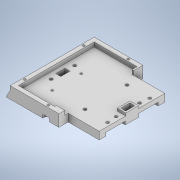
# Autodesk Inventor part: jeff
Saved by Autodesk Inventor 2020 (Build 240168000, 168)
## iProperties
Created: 2023-02-07
Part Number: jeff
Material: Generic
Document SubType Name: Modeling
Designer: user
Density: 1 g/cm^3
Appearance: Default
Author: user
Autodesk Inventor part; units mm, degrees
ref_plane "YZ Plane" through (0, 0, 0) normal (1, 0, 0) x (0, 1, 0)
ref_plane "XZ Plane" through (0, 0, 0) normal (0, 1, 0) x (-1, 0, 0)
ref_plane "XY Plane" through (0, 0, 0) normal (0, 0, 1) x (1, 0, 0)
sketch "Sketch1" plane through (0, 0, 0) normal (0, 1, 0) x (-1, 0, 0)
  line L0 (0, 0) -> (-100, 0)
  line L1 (-100, 0) -> (-100, -100)
  line L2 (-100, -100) -> (0, -100)
  line L3 (0, -100) -> (0, 0)
  dimension "d0" = 100
  dimension "d1" = 100
  constraints: 8 end point, 2 parallel, 1 horizontal, 1 perpendicular
  measures "d0" distance of L2.end L1.end
  measures "d1" distance of L1.end L0.end
extrude "base" add sketch "Sketch1" along normal blind 9
sketch "Sketch2" plane through (0, 9, 0) normal (0, 1, 0) x (1, 0, 0)
  circle A0 centre (96, 25) radius 1.75
  line L0 (100, 0) -> (100, 100) projected
  circle A1 centre (69, 25) radius 1.75
  line L1 (0, 0) -> (100, 0) projected
  line L2 (100, 50) -> (95, 50)
  circle A2 centre (96, 75) radius 1.75
  circle A3 centre (69, 75) radius 1.75
  line L3 (63, 0) -> (63, 100)
  line L4 (100, 100) -> (0, 100) projected
  line L5 (100, 25) -> (100, 11)
  line L6 (100, 11) -> (63, 11)
  line L7 (100, 89) -> (63, 89)
  circle A4 centre (82, 25) radius 17.5
  point P0 (63, 89)
  dimension "d6" = 4
  dimension "d7" = 3.5
  dimension "d9" = 3.5
  dimension "d10" = 27
  dimension "d11" = 25
  dimension "d13" = 37
  dimension "d14" = 14
  dimension "d17" = 35
  constraints: 10 end point, 5 centre point, 5 point on line, 4 symmetric about line, 1 horizontal, 1 horizontal alignment, 1 midpoint, 1 perpendicular, 1 vertical, 2 other
  measures "d6" distance from line of L0 A0.centre
  measures "d7" diameter of A0
  measures "d9" diameter of A1
  measures "d10" distance of A0.centre A1.centre
  measures "d11" distance from line of L1 A0.centre
  measures "d13" distance between parallel lines of L0 L3
  measures "d14" distance of L5.start L5.end
  measures "d17" diameter of A4
extrude "wheel space" cut sketch "Sketch2" against normal through all contours A0 | L1 L3 L6 A4 L0 | A4 L6 | L3 L4 L0 L7 | A1 | A2 | A3 picked at (84.4264, 10.3619)
sketch "Sketch3" plane through (0, 0, 0) normal (0, 0, 1) x (1, 0, 0)
  line L0 (63, 9) -> (0, 9) projected
  line L1 (0, 0) -> (0, 9) projected
  line L2 (63, 0) -> (0, 0) projected
  line L3 (5, 9) -> (0, 0)
  dimension "d18" = 5
  constraints: 2 end point, 1 point on line
  measures "d18" distance from line of L1 L3.start
extrude "ramp" cut sketch "Sketch3" against normal through all
sketch "Sketch4" plane through (0, 9, 0) normal (0, 1, 0) x (1, 0, 0)
  circle A0 centre (69, 75) radius 1.75 projected
  circle A1 centre (96, 25) radius 1.75 projected
  circle A2 centre (96, 75) radius 1.75 projected
  circle A3 centre (69, 25) radius 1.75 projected
  line L0 (5, 100) -> (5, 0) projected
  line L1 (5, 0) -> (63, 0) projected
  line L2 (63, 0) -> (63, 11) projected
  line L3 (63, 11) -> (100, 11) projected
  line L4 (100, 11) -> (100, 89) projected
  line L5 (100, 89) -> (63, 89) projected
  line L6 (63, 89) -> (63, 100) projected
  line L7 (63, 100) -> (5, 100) projected
  line L8 (63, 100) -> (63, 89) projected
  line L9 (61, 95) -> (10, 95)
  line L10 (10, 95) -> (10, 5)
  line L11 (10, 5) -> (63, 5)
  line L12 (63, 11) -> (63, 0) projected
  line L13 (63, 89) -> (61, 89)
  line L14 (61, 89) -> (61, 95)
  line L15 (63, 5) -> (53, 5)
  line L16 (53, 5) -> (53, 7)
  line L17 (53, 7) -> (63, 7)
  line L18 (63, 7) -> (63, 5)
  point P0 (0, 0)
  point P1 (63, 95)
  dimension "d21" = 5
  dimension "d22" = 5
  dimension "d23" = 5
  dimension "d64" = 2
  dimension "d72" = 10
  dimension "d73" = 2
  constraints: 18 end point, 5 perpendicular, 2 horizontal, 2 parallel, 1 point on line
  measures "d21" distance between parallel lines of L11 L1
  measures "d22" distance between parallel lines of L0 L10
  measures "d23" distance between parallel lines of L7 L9
  measures "d64" distance of L5.end L13.end
  measures "d72" distance of L16.end L17.end
  measures "d73" distance of L15.end L16.end
extrude "walls" add sketch "Sketch4" along normal blind 5 contours L7 L6 L13 L14 L9 L10 L11 L2 L1 L0 | L11 L16 L17 L2
sketch "Sketch5" plane through (0, 9, 0) normal (0, 1, 0) x (1, 0, 0)
  line L0 (22.7322, 84.5) -> (12.7322, 84.5)
  line L1 (12.7322, 84.5) -> (12.7322, 44.5)
  line L2 (12.7322, 44.5) -> (22.7322, 44.5)
  line L3 (22.7322, 44.5) -> (22.7322, 84.5)
  line L4 (14.7322, 44.5) -> (20.7322, 44.5)
  line L5 (20.7322, 44.5) -> (20.7322, 55.5)
  line L6 (20.7322, 55.5) -> (14.7322, 55.5)
  line L7 (14.7322, 55.5) -> (14.7322, 44.5)
  line L8 (14.7322, 44.5) -> (20.7322, 55.5) construction
  line L9 (20.7322, 44.5) -> (14.7322, 55.5) construction
  line L10 (10, 5) -> (10, 95) projected
  circle A0 centre (17.7322, 64) radius 1.75
  line L11 (100, 84.5) -> (90, 84.5)
  line L12 (90, 84.5) -> (90, 44.5)
  line L13 (90, 44.5) -> (100, 44.5)
  line L14 (100, 44.5) -> (100, 84.5)
  line L15 (92, 44.5) -> (98, 44.5)
  line L16 (98, 44.5) -> (98, 55.5)
  line L17 (98, 55.5) -> (92, 55.5)
  line L18 (92, 55.5) -> (92, 44.5)
  line L19 (92, 44.5) -> (98, 55.5) construction
  line L20 (98, 44.5) -> (92, 55.5) construction
  circle A1 centre (95, 64) radius 1.75
  circle A2 centre (96, 75) radius 1.75 projected
  line L21 (100, 11) -> (100, 89) projected
  circle A3 centre (95, 36) radius 1.75
  circle A4 centre (17.7322, 36) radius 1.75
  line L22 (100, 57.5) -> (90, 57.5)
  line L23 (90, 57.5) -> (90, 42.5)
  line L24 (90, 42.5) -> (100, 42.5)
  line L25 (100, 42.5) -> (100, 57.5)
  line L26 (100, 57.5) -> (90, 42.5) construction
  line L27 (90, 57.5) -> (100, 42.5) construction
  point P0 (0, 0)
  point P1 (17.7322, 50)
  point P2 (10, 50)
  point P3 (17.7322, 50)
  point P4 (95, 50)
  point P5 (95, 50)
  point P6 (95, 50)
  point P7 (17.7322, 50)
  point P8 (92, 44.5)
  point P9 (98, 44.5)
  point P10 (95, 84.5)
  dimension "d26" = 10
  dimension "d27" = 40
  dimension "d28" = 5.5
  dimension "d29" = 6
  dimension "d30" = 11
  dimension "d31" = 3.5
  dimension "d32" = 14
  dimension "d33" = 10
  dimension "d34" = 40
  dimension "d35" = 5.5
  dimension "d36" = 6
  dimension "d37" = 11
  dimension "d38" = 3.5
  dimension "d39" = 14
  dimension "d60" = 3.5
  dimension "d61" = 14
  dimension "d62" = 3.5
  dimension "d63" = 14
  dimension "d65" = 10
  dimension "d66" = 15
  constraints: 52 end point, 12 midpoint, 9 parallel, 5 horizontal, 5 perpendicular, 4 centre point, 1 collinear, 1 horizontal alignment, 1 vertical alignment
  measures "d26" distance of L2.end L1.end
  measures "d27" distance of L1.end L0.end
  measures "d28" distance from line of L2 point (17.732, 50)
  measures "d29" distance of L6.end L5.end
  measures "d30" distance of L5.end L4.end
  measures "d31" diameter of A0
  measures "d32" distance of point (17.732, 50) A0.centre
  measures "d33" distance of L14.start L12.end
  measures "d34" distance of L12.end L12.start
  measures "d35" distance from line of L13 point (95, 50)
  measures "d36" distance of L17.end L16.end
  measures "d37" distance of L16.end L15.end
  measures "d38" diameter of A1
  measures "d39" distance of point (95, 50) A1.centre
  measures "d60" diameter of A3
  measures "d61" distance of point (95, 50) A3.centre
  measures "d62" diameter of A4
  measures "d63" distance of A4.centre point (17.732, 50)
  measures "d65" distance of L24.end L23.end
  measures "d66" distance of L23.end L22.end
extrude "ir sensor" cut sketch "Sketch5" against normal through all contours L2 L7 L6 L5 | A0 | L13 L18 L17 L16 | A1 | A3 | A4
sketch "Sketch8" plane through (0, 14, 0) normal (0, 1, 0) x (1, 0, 0)
  line L0 (61, 89) -> (63, 89) projected
  line L1 (63, 89) -> (63, 100) projected
  line L2 (63, 100) -> (5, 100) projected
  line L3 (5, 100) -> (5, 0) projected
  line L4 (5, 0) -> (63, 0) projected
  line L5 (63, 0) -> (63, 7) projected
  line L6 (63, 7) -> (53, 7) projected
  line L7 (53, 7) -> (53, 5) projected
  line L8 (53, 5) -> (10, 5) projected
  line L9 (10, 5) -> (10, 95) projected
  line L10 (10, 95) -> (61, 95) projected
  line L11 (61, 95) -> (61, 89) projected
  circle A0 centre (7.5, 85) radius 1.25
  circle A1 centre (7.5, 15) radius 1.25
  circle A2 centre (48, 2.5) radius 1.25
  circle A3 centre (48, 97.5) radius 1.25
  point P0 (0, 0)
  dimension "d82" = 2.5
  dimension "d84" = 2.5
  dimension "d85" = 2.5
  dimension "d87" = 2.5
  dimension "d88" = 15
  dimension "d89" = 15
  dimension "d90" = 15
  dimension "d91" = 2.5
  dimension "d92" = 2.5
  dimension "d93" = 2.5
  constraints: 4 centre point, 2 vertical alignment
  measures "d82" diameter of A0
  measures "d84" diameter of A1
  measures "d85" diameter of A2
  measures "d87" diameter of A3
  measures "d88" distance from line of L2 A0.centre
  measures "d89" distance from line of L4 A1.centre
  measures "d90" distance from line of L1 A3.centre
  measures "d91" distance from line of L3 A0.centre
  measures "d92" distance from line of L10 A3.centre
  measures "d93" distance from line of L4 A2.centre
sketch "Sketch6" plane through (0, 9, 0) normal (0, 1, 0) x (1, 0, 0)
  line L0 (20.7322, 44.5) -> (14.7322, 44.5) projected
  circle A0 centre (17.7322, 64) radius 1.75 projected
  line L1 (53, 5) -> (10, 5) projected
  line L2 (10, 95) -> (61, 95) projected
  circle A1 centre (69, 25) radius 1.75 projected
  circle A2 centre (96, 25) radius 1.75 projected
  circle A3 centre (69, 25) radius 1.75 projected
  circle A4 centre (96, 25) radius 1.75 projected
  line L3 (69, 25) -> (96, 25)
  circle A5 centre (30, 25) radius 1.25
  line L4 (10, 5) -> (10, 95) projected
  circle A6 centre (30, 59.5) radius 1.25
  circle A7 centre (48, 97.5) radius 1.25 projected
  circle A8 centre (48, 2.5) radius 1.25 projected
  circle A9 centre (7.5, 85) radius 1.25 projected
  circle A10 centre (7.5, 15) radius 1.25 projected
  point P0 (0, 0)
  point P1 (63, 5)
  point P2 (63, 95)
  dimension "d75" = 2.5
  dimension "d76" = 20
  dimension "d77" = 20
  dimension "d79" = 2.5
  dimension "d80" = 34.5
  constraints: 2 centre point, 2 end point, 1 horizontal
  measures "d75" diameter of A5
  measures "d76" distance from line of L1 A5.centre
  measures "d77" distance from line of L4 A5.centre
  measures "d79" diameter of A6
  measures "d80" distance of A5.centre A6.centre
extrude "mount holes" cut sketch "Sketch6" against normal through all both and the other way through all contours A5 | A6 | A7 | A8 | A9 | A10
sketch "Sketch7" plane through (0, 0, 0) normal (0, -1, 0) x (1, 0, 0)
  line L0 (92, -44.5) -> (98, -44.5) projected
  line L1 (98, -44.5) -> (98, -55.5) projected
  line L2 (98, -55.5) -> (92, -55.5) projected
  line L3 (92, -55.5) -> (92, -44.5) projected
  circle A0 centre (17.7322, -64) radius 1.75 projected
  circle A1 centre (95, -64) radius 1.75 projected
  line L4 (20.7322, -44.5) -> (20.7322, -55.5) projected
  line L5 (20.7322, -55.5) -> (14.7322, -55.5) projected
  line L6 (14.7322, -55.5) -> (14.7322, -44.5) projected
  line L7 (14.7322, -44.5) -> (20.7322, -44.5) projected
  circle A2 centre (69, -75) radius 1.75 projected
  circle A3 centre (96, -25) radius 1.75 projected
  circle A4 centre (96, -75) radius 1.75 projected
  circle A5 centre (69, -25) radius 1.75 projected
  line L8 (63, -100) -> (63, -89) projected
  line L9 (63, -89) -> (100, -89) projected
  line L10 (100, -11) -> (100, -89) projected
  line L11 (100, -11) -> (63, -11) projected
  line L12 (63, -11) -> (63, 0) projected
  line L13 (0, 0) -> (63, 0) projected
  line L14 (0, -100) -> (0, 0) projected
  line L15 (63, -100) -> (0, -100) projected
  circle A6 centre (69, -75) radius 6
  circle A7 centre (69, -25) radius 1.75 projected
  circle A8 centre (69, -25) radius 6
  circle A9 centre (96, -25) radius 1.75 projected
  circle A10 centre (17.7322, -64) radius 6
  circle A11 centre (95, -36) radius 1.75 projected
  arc A12 (89, -36) -> (95, -42) centre (95, -36) ccw
  line L16 (98, -31) -> (98.3166, -31)
  line L17 (100, -11) -> (100, -89) projected
  line L18 (96, -19) -> (100, -19)
  line L19 (100, -50) -> (98.3161, -50)
  line L20 (95, -42) -> (100, -42)
  circle A13 centre (17.7322, -36) radius 1.75 projected
  circle A14 centre (17.7322, -36) radius 6
  line L21 (92, -19) -> (96, -19)
  line L22 (89, -36) -> (89, -19)
  line L23 (89, -19) -> (92, -19)
  circle A15 centre (96, -75) radius 1.75
  circle A16 centre (96, -75) radius 1.75
  circle A17 centre (95, -64) radius 1.75
  arc A18 (95, -58) -> (89, -64) centre (95, -64) ccw
  line L24 (98, -69) -> (98.3166, -69)
  line L25 (96, -81) -> (100, -81)
  line L26 (95, -58) -> (100, -58)
  line L27 (92, -81) -> (96, -81)
  line L28 (89, -64) -> (89, -81)
  line L29 (89, -81) -> (92, -81)
  circle A19 centre (30, -59.5) radius 1.25 projected
  circle A20 centre (30, -25) radius 1.25 projected
  circle A21 centre (30, -59.5) radius 6
  circle A22 centre (30, -25) radius 6
  circle A23 centre (48, -97.5) radius 1.25 projected
  circle A24 centre (48, -2.5) radius 1.25 projected
  circle A25 centre (7.5, -15) radius 1.25 projected
  circle A26 centre (7.5, -85) radius 1.25 projected
  arc A27 (52, -97.5) -> (44, -97.5) centre (48, -97.5) ccw
  line L30 (44, -97.5) -> (44, -100)
  line L31 (63, -100) -> (5, -100) projected
  line L32 (52, -97.5) -> (52, -100)
  line L33 (44, -2.5) -> (44, 0)
  line L34 (0, 0) -> (63, 0) projected
  line L35 (52, -2.5) -> (52, 0)
  circle A28 centre (7.5, -15) radius 4
  circle A29 centre (7.5, -85) radius 4
  arc A30 (44, -2.5) -> (52, -2.5) centre (48, -2.5) ccw
  point P0 (100, -31)
  point P1 (96, -31)
  point P2 (93.1644, -30.2877)
  point P3 (96, -69)
  point P4 (93.1644, -69.7123)
  dimension "d69" = 12
  dimension "d71" = 12
  dimension "d94" = 8
  dimension "d96" = 8
  dimension "d97" = 8
  constraints: 34 end point, 15 centre point, 15 symmetric about line, 12 coincident, 10 point on circle, 9 point on line, 5 equal radius, 5 perpendicular, 3 tangent, 2 equal length, 2 horizontal, 2 vertical, 1 midpoint, 4 other
  measures "d69" diameter of A12
  measures "d71" diameter of A8
  measures "d94" diameter of A27
  measures "d96" diameter of A28
  measures "d97" diameter of A29
extrude "mount holes flush" cut sketch "Sketch7" against normal blind 4 contours L15 L30 A27 L32 | L25 L27 L29 L28 A18 L26 L10 | L20 A12 L22 L23 L21 L18 L10 | L13 L35 A30 L33 | A6 | A8 | A10 | A14 | A20 | A21 | A22 | A28 | A29
extrude "Extrusion8" add sketch "Sketch5" along normal blind 3 contours L14 L13 L16 L17 L18 L12 L22 | L21 L24 L23 L13
body "Solid1"
